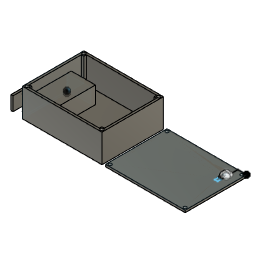
Cadeadov1.0 v4-Tampa (Autodesk Fusion 360 design; units mm, degrees)
Autodesk Fusion 360 part; units mm, degrees
note: some values were not read from the file. Set by a fixed rule: which sketch regions a step uses.
sketch "Sketch1" plane through (0, 0, 0) normal (0, 0, 1) x (1, 0, 0)
  line L0 (0, 0) -> (110, 0)
  line L1 (110, 0) -> (110, 85)
  line L2 (110, 85) -> (0, 85)
  line L3 (0, 85) -> (0, 0)
  dimension "d1" = 110
  dimension "d2" = 85
  constraint horizontal L0
  constraint vertical L1
  constraint horizontal L2
  constraint vertical L3
  constraint coincident L0.start L3.end
  measures "d1" distance of L0.start L0.end
  measures "d2" distance of L0.start L2.end
extrude "Extrude1" add sketch "Sketch1" along normal blind 3 makes body 1
sketch "Sketch2" plane through (0, 0, 3) normal (0, 0, 1) x (-1, 0, 0)
  line L0 (0, -85) -> (0, 0)
  line L1 (0, 0) -> (-110, 0)
  line L2 (-110, 0) -> (-110, -85)
  line L3 (-110, -85) -> (0, -85)
  line L4 (0, 0) -> (-6.5, 0)
  line L5 (-6.5, 0) -> (-6.5, -6.5)
  line L6 (-6.5, -6.5) -> (0, -6.5)
  line L7 (0, -6.5) -> (0, 0)
  line L8 (0, -85) -> (-6.5, -85)
  line L9 (-6.5, -85) -> (-6.5, -78.5)
  line L10 (-6.5, -78.5) -> (0, -78.5)
  line L11 (0, -78.5) -> (0, -85)
  line L12 (-110, -85) -> (-103.5, -85)
  line L13 (-103.5, -85) -> (-103.5, -78.5)
  line L14 (-103.5, -78.5) -> (-110, -78.5)
  line L15 (-110, -78.5) -> (-110, -85)
  line L16 (-110, 0) -> (-103.5, 0)
  line L17 (-103.5, 0) -> (-103.5, -6.5)
  line L18 (-103.5, -6.5) -> (-110, -6.5)
  line L19 (-110, -6.5) -> (-110, 0)
  line L20 (-6.5, 0) -> (-103.5, 0)
  line L21 (-103.5, 0) -> (-103.5, -3)
  line L22 (-103.5, -3) -> (-6.5, -3)
  line L23 (-6.5, -3) -> (-6.5, 0)
  line L24 (-110, -6.5) -> (-107, -6.5)
  line L25 (-107, -6.5) -> (-107, -78.5)
  line L26 (-107, -78.5) -> (-110, -78.5)
  line L27 (-110, -78.5) -> (-110, -6.5)
  line L28 (-103.5, -85) -> (-6.5, -85)
  line L29 (-6.5, -85) -> (-6.5, -82)
  line L30 (-6.5, -82) -> (-103.5, -82)
  line L31 (-103.5, -82) -> (-103.5, -85)
  line L32 (0, -78.5) -> (-3, -78.5)
  line L33 (-3, -78.5) -> (-3, -6.5)
  line L34 (-3, -6.5) -> (0, -6.5)
  line L35 (0, -6.5) -> (0, -78.5)
  dimension "d5" = 6.5
  dimension "d6" = 6.5
  dimension "d7" = 6.5
  dimension "d8" = 6.5
  dimension "d9" = 6.5
  dimension "d10" = 6.5
  dimension "d11" = 6.5
  dimension "d12" = 6.5
  dimension "d13" = 97
  dimension "d14" = 3
  dimension "d15" = 3
  dimension "d16" = 72
  dimension "d17" = 3
  dimension "d18" = 3
  constraint horizontal L4
  constraint vertical L5
  constraint horizontal L6
  constraint vertical L7
  constraint coincident L0.end L1.start
  constraint horizontal L8
  constraint vertical L9
  constraint horizontal L10
  constraint vertical L11
  constraint coincident L0.start L3.end
  constraint horizontal L12
  constraint vertical L13
  constraint horizontal L14
  constraint vertical L15
  constraint coincident L2.end L3.start
  constraint horizontal L16
  constraint vertical L17
  constraint horizontal L18
  constraint vertical L19
  constraint coincident L1.end L2.start
  constraint horizontal L20
  constraint vertical L21
  constraint horizontal L22
  constraint vertical L23
  constraint horizontal L24
  constraint vertical L25
  constraint horizontal L26
  constraint vertical L27
  constraint horizontal L28
  constraint vertical L29
  constraint horizontal L30
  constraint vertical L31
  constraint horizontal L32
  constraint vertical L33
  constraint horizontal L34
  constraint vertical L35
  constraint coincident L6 L33.end
  measures "d5" distance of L0.end L4.end
  measures "d6" distance of L0.end L6.end
  measures "d7" distance of L0.start L8.end
  measures "d8" distance of L0.start L10.end
  measures "d9" distance of L2.end L12.end
  measures "d10" distance of L2.end L14.end
  measures "d11" distance of L1.end L16.end
  measures "d12" distance of L1.end L18.end
  measures "d13" distance of L4.end L16.end
  measures "d14" distance of L4.end L22.end
  measures "d15" distance of L18.end L24.end
  measures "d16" distance of L18.end L14.end
  measures "d17" distance of L12.end L30.end
  measures "d18" distance of L10.end L32.end
extrude "Extrude2" add sketch "Sketch2" along normal blind 36 contours L0 L3 L8 L9 L10 L11 L29 L32 | L0 L6 L10 L32 L33 L34 L35 | L3 L9 L13 L28 L29 L30 L31 | L0 L1 L4 L5 L6 L7 L23 L34 | L2 L3 L12 L13 L14 L15 L26 L31 | L1 L5 L17 L20 L21 L22 L23 | L2 L14 L18 L24 L25 L26 L27 | L1 L2 L16 L17 L18 L19 L21 L24 bodies 1
sketch "Sketch3" plane through (0, 0, 3) normal (0, 0, 1) x (-1, 0, 0)
  line L0 (-6.5, -78.5) -> (-3, -78.5)
  line L1 (-3, -78.5) -> (-3, -6.5)
  line L2 (-3, -6.5) -> (-6.5, -6.5)
  line L3 (-6.5, -6.5) -> (-6.5, -3)
  line L4 (-6.5, -3) -> (-103.5, -3)
  line L5 (-103.5, -3) -> (-103.5, -6.5)
  line L6 (-103.5, -6.5) -> (-107, -6.5)
  line L7 (-107, -6.5) -> (-107, -78.5)
  line L8 (-107, -78.5) -> (-103.5, -78.5)
  line L9 (-103.5, -78.5) -> (-103.5, -82)
  line L10 (-103.5, -82) -> (-6.5, -82)
  line L11 (-6.5, -82) -> (-6.5, -78.5)
  line L12 (-6.5, -3) -> (-33.5, -3)
  line L13 (-6.5, -6.5) -> (-6.5, -61.5)
  line L14 (-6.5, -61.5) -> (-1.333, -61.5)
  line L15 (-3, -61.5) -> (-36.5, -61.5)
  line L16 (-36.5, -61.5) -> (-36.5, -64.5)
  line L17 (-36.5, -64.5) -> (-3, -64.5)
  line L18 (-3, -64.5) -> (-3, -61.5)
  line L19 (-36.5, -64.5) -> (-33.5, -64.5)
  line L20 (-33.5, -64.5) -> (-33.5, -3)
  line L21 (-33.5, -3) -> (-36.5, -3)
  line L22 (-36.5, -3) -> (-36.5, -64.5)
  dimension "d21" = 27
  dimension "d22" = 55
  dimension "d23" = 33.5
  dimension "d24" = 3
  constraint coincident L3.end L4.start
  constraint perpendicular L3 L12
  constraint coincident L2.end L3.start
  constraint perpendicular L2 L13
  constraint perpendicular L1 L14
  constraint horizontal L15
  constraint vertical L16
  constraint horizontal L17
  constraint vertical L18
  constraint coincident L14 L15.start
  constraint coincident L1 L15.start
  constraint horizontal L19
  constraint vertical L20
  constraint horizontal L21
  constraint vertical L22
  measures "d21" distance of L3.end L12.end
  measures "d22" distance of L2.end L13.end
  measures "d23" distance of L15.start L15.end
  measures "d24" distance of L15.start L17.end
extrude "Extrude3" add sketch "Sketch3" along normal blind 20.5 contours L1 L14 L15 L17 L18 L20 | L15 L16 L17 L19 L20 L22 | L4 L15 L20 L21 L22 bodies 1
sketch "Sketch4" plane through (0, 0, 23.5) normal (0, 0, 1) x (-1, 0, 0)
  line L0 (-36.5, -3) -> (-36.5, -64.5)
  line L1 (-36.5, -64.5) -> (-3, -64.5)
  line L2 (-3, -64.5) -> (-3, -61.5)
  line L3 (-3, -61.5) -> (-33.5, -61.5)
  line L4 (-33.5, -61.5) -> (-33.5, -3)
  line L5 (-33.5, -3) -> (-36.5, -3)
  line L6 (-3, -64.5) -> (-36.5, -64.5)
  line L7 (-36.5, -64.5) -> (-36.5, -3)
  line L8 (-36.5, -3) -> (-3, -3)
  line L9 (-3, -3) -> (-3, -64.5)
  constraint horizontal L6
  constraint vertical L7
  constraint horizontal L8
  constraint vertical L9
  constraint coincident L0.start L5.end
  constraint coincident L1.end L2.start
sketch "Sketch5" plane through (0, 0, 23.5) normal (0, 0, 1) x (1, 0, 0)
sketch "Sketch6" plane through (0, 0, 23.5) normal (0, 0, 1) x (1, 0, 0)
sketch "Sketch7" plane through (0, 0, 23.5) normal (0, 0, 1) x (-1, 0, 0)
extrude "Extrude4" add sketch "Sketch4" along normal blind 3 contours L0 L1 L2 L3 L4 L5 L6 L7 L8 L9 bodies 1
sketch "Sketch8" plane through (0, 61.5, 0) normal (0, -1, 0) x (1, 0, 0)
  line L0 (3, 3) -> (33.5, 3)
  line L1 (33.5, 3) -> (33.5, 26.5)
  line L2 (33.5, 26.5) -> (3, 26.5)
  line L3 (3, 26.5) -> (3, 3)
  line L4 (3, 26.5) -> (33.5, 26.5)
  line L5 (33.5, 26.5) -> (33.5, 23.5)
  line L6 (33.5, 23.5) -> (3, 23.5)
  line L7 (3, 23.5) -> (3, 26.5)
  dimension "d29" = 3
  constraint horizontal L4
  constraint vertical L5
  constraint horizontal L6
  constraint vertical L7
  constraint coincident L2.end L3.start
  measures "d29" distance of L2.end L6.end
extrude "Extrude5" add sketch "Sketch8" along normal blind 55 contours L1 L2 L3 L4 L5 L6 L7 bodies 1
sketch "Sketch9" plane through (33.5, 0, 0) normal (-1, 0, 0) x (0, -1, 0)
  line L0 (-6.5, 23.5) -> (-61.5, 23.5)
  line L1 (-61.5, 23.5) -> (-61.5, 3)
  line L2 (-61.5, 3) -> (-3, 3)
  line L3 (-3, 3) -> (-3, 26.5)
  line L4 (-3, 26.5) -> (-6.5, 26.5)
  line L5 (-6.5, 26.5) -> (-6.5, 23.5)
  line L6 (-6.5, 26.5) -> (-3, 26.5)
  line L7 (-3, 26.5) -> (-3, 23.5)
  line L8 (-3, 23.5) -> (-6.5, 23.5)
  line L9 (-6.5, 23.5) -> (-6.5, 26.5)
  dimension "d32" = 3
  constraint horizontal L6
  constraint vertical L7
  constraint horizontal L8
  constraint vertical L9
  constraint coincident L4.end L5.start
  measures "d32" distance of L4.end L0.start
extrude "Extrude6" add sketch "Sketch9" along normal blind 27 contours L3 L4 L5 L6 L7 L8 L9 bodies 1
sketch "Sketch10" plane through (0, 0, 0) normal (-1, 0, 0) x (0, -1, 0)
  line L0 (-85, 0) -> (0, 0)
  line L1 (0, 0) -> (0, 39)
  line L2 (0, 39) -> (-85, 39)
  line L3 (-85, 39) -> (-85, 0)
  line L4 (0, 0) -> (-6.5, 0)
  line L5 (-6.5, 0) -> (-6.5, 3)
  line L6 (-6.5, 3) -> (-6.5, 23.5)
  line L7 (-6.5, 23.5) -> (-61.5, 23.5)
  line L8 (-61.5, 23.5) -> (-61.5, 3)
  line L9 (-61.5, 3) -> (-6.5, 3)
  dimension "d35" = 6.5
  dimension "d36" = 3
  dimension "d37" = 20.5
  dimension "d38" = 55
  constraint coincident L0.end L1.start
  constraint perpendicular L1 L4
  constraint perpendicular L4 L5
  constraint perpendicular L0 L6
  constraint perpendicular L6 L7
  constraint perpendicular L0 L8
  constraint perpendicular L5 L9
  measures "d35" distance of L0.end L4.end
  measures "d36" distance of L4.end L5.end
  measures "d37" distance of L5.end L6.end
  measures "d38" distance of L6.end L7.end
extrude "Extrude7" cut sketch "Sketch10" against normal blind 3 contours L6 L7 L8 L9 bodies 1
sketch "Sketch11" plane through (0, 0, 39) normal (0, 0, 1) x (-1, 0, 0)
  line L0 (-6.5, -78.5) -> (-6.5, -82)
  line L1 (-6.5, -82) -> (-103.5, -82)
  line L2 (-103.5, -82) -> (-103.5, -78.5)
  line L3 (-103.5, -78.5) -> (-107, -78.5)
  line L4 (-107, -78.5) -> (-107, -6.5)
  line L5 (-107, -6.5) -> (-103.5, -6.5)
  line L6 (-103.5, -6.5) -> (-103.5, -3)
  line L7 (-103.5, -3) -> (-6.5, -3)
  line L8 (-6.5, -3) -> (-6.5, -6.5)
  line L9 (-6.5, -6.5) -> (-3, -6.5)
  line L10 (-3, -6.5) -> (-3, -78.5)
  line L11 (-3, -78.5) -> (-6.5, -78.5)
  line L12 (0, 0) -> (-110, 0)
  line L13 (-110, 0) -> (-110, -85)
  line L14 (-110, -85) -> (0, -85)
  line L15 (0, -85) -> (0, 0)
  line L16 (0, -78.5) -> (-3.25, -78.5)
  line L17 (-3.25, -78.5) -> (-3.25, -81.75)
  circle A0 centre (-3.25, -81.75) radius 2.2
  line L18 (0, 0) -> (-3.25, 0)
  line L19 (-3.25, 0) -> (-3.25, -3.25)
  circle A1 centre (-3.25, -3.25) radius 2.2
  line L20 (-110, 0) -> (-106.75, 0)
  line L21 (-106.75, 0) -> (-106.75, -3.25)
  circle A2 centre (-106.75, -3.25) radius 2.2
  line L22 (-110, -85) -> (-106.75, -85)
  line L23 (-106.75, -85) -> (-106.75, -81.75)
  circle A3 centre (-106.75, -81.75) radius 2.2
  dimension "d41" = 3.25
  dimension "d42" = 3.25
  dimension "d43" = 4.4
  dimension "d44" = 3.25
  dimension "d45" = 3.25
  dimension "d46" = 4.4
  dimension "d47" = 3.25
  dimension "d48" = 3.25
  dimension "d49" = 4.4
  dimension "d50" = 3.25
  dimension "d51" = 3.25
  dimension "d52" = 4.4
  constraint coincident L15 L16.start
  constraint perpendicular L10 L16
  constraint perpendicular L14 L17
  constraint coincident L17.end A0.centre
  constraint coincident L12.start L15.end
  constraint perpendicular L15 L18
  constraint perpendicular L12 L19
  constraint coincident L19.end A1.centre
  constraint coincident L12.end L13.start
  constraint perpendicular L13 L20
  constraint perpendicular L20 L21
  constraint coincident L21.end A2.centre
  constraint coincident L13.end L14.start
  constraint perpendicular L13 L22
  constraint perpendicular L22 L23
  constraint coincident L23.end A3.centre
  measures "d41" distance of L16.start L16.end
  measures "d42" distance of L16.end L17.end
  measures "d43" diameter of A0
  measures "d44" distance of L12.start L18.end
  measures "d45" distance of L18.end L19.end
  measures "d46" diameter of A1
  measures "d47" distance of L12.end L20.end
  measures "d48" distance of L20.end L21.end
  measures "d49" diameter of A2
  measures "d50" distance of L13.end L22.end
  measures "d51" distance of L22.end L23.end
  measures "d52" diameter of A3
extrude "Extrude8" cut sketch "Sketch11" against normal blind 15 contours A0 | A1 | A2 | A3 bodies 1
sketch "Sketch12" plane through (0, 0, 0) normal (0, 0, 1) x (1, 0, 0)
  line L0 (115, 0) -> (225, 0)
  line L1 (225, 0) -> (225, 85)
  line L2 (225, 85) -> (115, 85)
  line L3 (115, 85) -> (115, 0)
  dimension "d55" = 110
  dimension "d56" = 85
  constraint horizontal L0
  constraint vertical L1
  constraint horizontal L2
  constraint vertical L3
  measures "d55" distance of L0.start L0.end
  measures "d56" distance of L0.start L2.end
extrude "Extrude9" add sketch "Sketch12" along normal blind 3 separate body makes body 2
sketch "Sketch13" plane through (0, 0, 3) normal (0, 0, 1) x (-1, 0, 0)
  line L0 (-115, -85) -> (-115, 0)
  line L1 (-115, 0) -> (-225, 0)
  line L2 (-225, 0) -> (-225, -85)
  line L3 (-225, -85) -> (-115, -85)
  line L4 (-115, 0) -> (-118.25, 0)
  line L5 (-118.25, 0) -> (-118.25, -3.25)
  circle A0 centre (-118.25, -3.25) radius 2.2
  line L6 (-115, -85) -> (-118.25, -85)
  line L7 (-118.25, -85) -> (-118.25, -81.75)
  circle A1 centre (-118.25, -81.75) radius 2.2
  line L8 (-225, -85) -> (-221.75, -85)
  line L9 (-221.75, -85) -> (-221.75, -81.75)
  circle A2 centre (-221.75, -81.75) radius 2.2
  line L10 (-225, 0) -> (-221.75, 0)
  line L11 (-221.75, 0) -> (-221.75, -3.25)
  circle A3 centre (-221.75, -3.25) radius 2.2
  circle A4 centre (-118.25, -81.75) radius 2.1
  circle A5 centre (-221.75, -81.75) radius 2.1
  circle A6 centre (-221.75, -3.25) radius 2.1
  circle A7 centre (-118.25, -3.25) radius 2.1
  dimension "d59" = 3.25
  dimension "d60" = 3.25
  dimension "d61" = 4.4
  dimension "d62" = 3.25
  dimension "d63" = 3.25
  dimension "d64" = 4.4
  dimension "d65" = 3.25
  dimension "d66" = 3.25
  dimension "d67" = 4.4
  dimension "d68" = 3.25
  dimension "d69" = 3.25
  dimension "d70" = 4.4
  dimension "d71" = 4.2
  dimension "d72" = 4.2
  dimension "d73" = 4.2
  dimension "d74" = 4.2
  constraint coincident L0.end L1.start
  constraint perpendicular L0 L4
  constraint perpendicular L4 L5
  constraint coincident L5.end A0.centre
  constraint coincident L0.start L3.end
  constraint perpendicular L0 L6
  constraint perpendicular L6 L7
  constraint coincident L7.end A1.centre
  constraint coincident L2.end L3.start
  constraint perpendicular L2 L8
  constraint perpendicular L8 L9
  constraint coincident L9.end A2.centre
  constraint coincident L1.end L2.start
  constraint perpendicular L2 L10
  constraint perpendicular L10 L11
  constraint coincident L11.end A3.centre
  constraint concentric A1 A4
  constraint concentric A2 A5
  constraint concentric A3 A6
  constraint concentric A0 A7
  measures "d59" distance of L0.end L4.end
  measures "d60" distance of L4.end L5.end
  measures "d61" diameter of A0
  measures "d62" distance of L0.start L6.end
  measures "d63" distance of L6.end L7.end
  measures "d64" diameter of A1
  measures "d65" distance of L2.end L8.end
  measures "d66" distance of L8.end L9.end
  measures "d67" diameter of A2
  measures "d68" distance of L1.end L10.end
  measures "d69" distance of L10.end L11.end
  measures "d70" diameter of A3
  measures "d71" diameter of A4
  measures "d72" diameter of A5
  measures "d73" diameter of A6
  measures "d74" diameter of A7
extrude "Extrude10" cut sketch "Sketch13" against normal blind 3 contours A4 | A5 | A6 | A7 bodies 2
sketch "Sketch14" plane through (0, 61.5, 0) normal (0, -1, 0) x (1, 0, 0)
  line L0 (33.5, 23.5) -> (0, 23.5)
  line L1 (0, 23.5) -> (0, 3)
  line L2 (0, 3) -> (33.5, 3)
  line L3 (33.5, 3) -> (33.5, 23.5)
  line L4 (0, 3) -> (3, 3)
  line L5 (3, 3) -> (3, 6)
  line L6 (3, 6) -> (0, 6)
  line L7 (0, 6) -> (0, 3)
  constraint horizontal L4
  constraint vertical L5
  constraint horizontal L6
  constraint vertical L7
  constraint coincident L1.end L2.start
sketch "Sketch15" plane through (0, 61.5, 0) normal (0, -1, 0) x (1, 0, 0)
  line L0 (0, 6) -> (3, 6)
  line L1 (3, 6) -> (3, 9)
  line L2 (3, 9) -> (0, 9)
  line L3 (0, 9) -> (0, 6)
  constraint horizontal L0
  constraint vertical L1
  constraint horizontal L2
  constraint vertical L3
extrude "Extrude11" cut sketch "Sketch15" against normal blind 3 bodies 1
sketch "Sketch16" plane through (16.75, 61.5, 13.25) normal (0, -1, 0) x (1, 0, 0)
sketch "Sketch17" plane through (16.75, 61.5, 13.25) normal (0, -1, 0) x (1, 0, 0)
sketch "Sketch18" plane through (0, 0, 0) normal (-1, 0, 0) x (0, -1, 0)
  line L0 (-85, 0) -> (0, 0)
  line L1 (0, 0) -> (0, 39)
  line L2 (0, 39) -> (-85, 39)
  line L3 (-85, 39) -> (-85, 0)
  line L4 (-61.5, 6) -> (-64.5, 6)
  line L5 (-64.5, 6) -> (-64.5, 9)
  line L6 (-64.5, 9) -> (-61.5, 9)
  line L7 (-61.5, 9) -> (-61.5, 23.5)
  line L8 (-61.5, 23.5) -> (-6.5, 23.5)
  line L9 (-6.5, 23.5) -> (-6.5, 3)
  line L10 (-6.5, 3) -> (-61.5, 3)
  line L11 (-61.5, 3) -> (-61.5, 6)
  line L12 (-64.5, 9) -> (-61.5, 9)
  line L13 (-61.5, 9) -> (-61.5, 12)
  line L14 (-61.5, 12) -> (-64.5, 12)
  line L15 (-64.5, 12) -> (-64.5, 9)
  line L16 (-61.5, 12) -> (-64.5, 12)
  line L17 (-64.5, 12) -> (-64.5, 15)
  line L18 (-64.5, 15) -> (-61.5, 15)
  line L19 (-61.5, 15) -> (-61.5, 12)
  constraint horizontal L12
  constraint vertical L13
  constraint horizontal L14
  constraint vertical L15
  constraint coincident L7 L13.end
  constraint coincident L5.end L6.start
  constraint horizontal L16
  constraint vertical L17
  constraint horizontal L18
  constraint vertical L19
extrude "Extrude12" cut sketch "Sketch18" against normal blind 3 contours L7 L14 L16 L17 L18 L19 bodies 1
sketch "Sketch19" plane through (0, 0, 0) normal (-1, 0, 0) x (0, -1, 0)
  line L0 (-64.5, 15) -> (-61.5, 15)
  line L1 (-61.5, 15) -> (-61.5, 23.5)
  line L2 (-61.5, 23.5) -> (-6.5, 23.5)
  line L3 (-6.5, 23.5) -> (-6.5, 3)
  line L4 (-6.5, 3) -> (-61.5, 3)
  line L5 (-61.5, 3) -> (-61.5, 6)
  line L6 (-61.5, 6) -> (-64.5, 6)
  line L7 (-64.5, 6) -> (-64.5, 9)
  line L8 (-64.5, 9) -> (-61.5, 9)
  line L9 (-61.5, 9) -> (-61.5, 12)
  line L10 (-61.5, 12) -> (-64.5, 12)
  line L11 (-64.5, 12) -> (-64.5, 15)
  line L12 (-85, 0) -> (0, 0)
  line L13 (0, 0) -> (0, 39)
  line L14 (0, 39) -> (-85, 39)
  line L15 (-85, 39) -> (-85, 0)
  line L16 (-61.5, 15) -> (-64.5, 15)
  line L17 (-64.5, 15) -> (-64.5, 18)
  line L18 (-64.5, 18) -> (-61.5, 18)
  line L19 (-61.5, 18) -> (-61.5, 15)
  line L20 (-61.5, 18) -> (-64.5, 18)
  line L21 (-64.5, 18) -> (-64.5, 21)
  line L22 (-64.5, 21) -> (-61.5, 21)
  line L23 (-61.5, 21) -> (-61.5, 18)
  dimension "d81" = 3
  dimension "d82" = 3
  dimension "d83" = 3
  dimension "d84" = 3
  constraint horizontal L16
  constraint vertical L17
  constraint horizontal L18
  constraint vertical L19
  constraint coincident L0.end L1.start
  constraint horizontal L20
  constraint vertical L21
  constraint horizontal L22
  constraint vertical L23
  measures "d81" distance of L0.end L0.start
  measures "d82" distance of L0.end L18.end
  measures "d83" distance of L18.end L17.end
  measures "d84" distance of L18.end L22.end
extrude "Extrude13" cut sketch "Sketch19" against normal blind 3 contours L1 L18 L20 L21 L22 L23 bodies 1
sketch "Sketch20" plane through (0, 0, 0) normal (0, 0, 1) x (1, 0, 0)
  line L0 (-15, 2) -> (-18, 2)
  line L1 (-18, 2) -> (-18, 60)
  line L2 (-18, 60) -> (-15, 60)
  line L3 (-15, 60) -> (-15, 2)
  line L4 (-18, 60) -> (-15, 60)
  line L5 (-15, 60) -> (-15, 57)
  line L6 (-15, 57) -> (-18, 57)
  line L7 (-18, 57) -> (-18, 60)
  circle A0 centre (-16.5, 58.5) radius 1.5
  dimension "d87" = 3
  dimension "d88" = 58
  dimension "d89" = 3
  dimension "d90" = 3
  constraint horizontal L0
  constraint vertical L1
  constraint horizontal L2
  constraint vertical L3
  constraint horizontal L4
  constraint vertical L5
  constraint horizontal L6
  constraint vertical L7
  constraint tangent L3 A0
  measures "d87" distance of L0.start L0.end
  measures "d88" distance of L0.start L2.end
  measures "d89" distance of L1.end L2.end
  measures "d90" distance of L1.end L6.end
extrude "Extrude14" add sketch "Sketch20" along normal blind 20 separate body contours L0 L1 L3 L6 | L3 L5 L6 A0 | L1 L6 L7 A0 | A0 makes body 3
extrude "Extrude15" cut 1 faces at (-17, 38.6667, 20) along direction (0, 0, -1) blind 1 on bodies 3 bodies 3
sketch "Sketch21" plane through (-18, 0, 0) normal (-1, 0, 0) x (0, -1, 0)
  line L0 (-2, 19) -> (-58.5, 19)
  line L1 (-58.5, 19) -> (-58.5, 0)
  line L2 (-58.5, 0) -> (-2, 0)
  line L3 (-2, 0) -> (-2, 19)
  line L4 (-60, 0) -> (-57, 0)
  line L5 (-57, 0) -> (-57, 2.25)
  line L6 (-57, 2.25) -> (-60, 2.25)
  line L7 (-60, 2.25) -> (-60, 0)
  line L8 (-57, 2.25) -> (-60, 2.25)
  line L9 (-60, 2.25) -> (-60, 5.15)
  line L10 (-60, 5.15) -> (-57, 5.15)
  line L11 (-57, 5.15) -> (-57, 2.25)
  dimension "d95" = 3
  dimension "d96" = 2.25
  dimension "d97" = 2.9
  constraint horizontal L4
  constraint vertical L5
  constraint horizontal L6
  constraint vertical L7
  constraint horizontal L8
  constraint vertical L9
  constraint horizontal L10
  constraint vertical L11
  measures "d95" distance of L4.start L4.end
  measures "d96" distance of L4.start L6.end
  measures "d97" distance of L5.end L10.end
sketch "Sketch22" plane through (-18, 30.25, 9.5) normal (-1, 0, 0) x (0, -1, 0)
extrude "Extrude16" cut sketch "Sketch21" against normal blind 4 contours L1 L2 L4 L5 L6 L8 | L1 L4 L6 L7 L8 bodies 3
sketch "Sketch23" plane through (-18, 0, 0) normal (-1, 0, 0) x (0, -1, 0)
  line L0 (-57, 2.25) -> (-57, 0)
  line L1 (-57, 0) -> (-2, 0)
  line L2 (-2, 0) -> (-2, 19)
  line L3 (-2, 19) -> (-58.5, 19)
  line L4 (-58.5, 19) -> (-58.5, 2.25)
  line L5 (-58.5, 2.25) -> (-57, 2.25)
  line L6 (-57, 2.25) -> (-60, 2.25)
  line L7 (-60, 2.25) -> (-60, 5.15)
  line L8 (-60, 5.15) -> (-57, 5.15)
  line L9 (-57, 5.15) -> (-57, 2.25)
  line L10 (-57, 5.15) -> (-59.9423, 5.15)
  line L11 (-59.9423, 5.15) -> (-59.9423, 8.3)
  line L12 (-59.9423, 8.3) -> (-57, 8.3)
  line L13 (-57, 8.3) -> (-57, 5.15)
  line L14 (-57, 8.3) -> (-60, 8.3)
  line L15 (-60, 8.3) -> (-60, 11.2)
  line L16 (-60, 11.2) -> (-57, 11.2)
  line L17 (-57, 11.2) -> (-57, 8.3)
  line L18 (-57, 11.2) -> (-60, 11.2)
  line L19 (-60, 11.2) -> (-60, 14.25)
  line L20 (-60, 14.25) -> (-57, 14.25)
  line L21 (-57, 14.25) -> (-57, 11.2)
  line L22 (-57, 14.25) -> (-60, 14.25)
  line L23 (-60, 14.25) -> (-60, 17.15)
  line L24 (-60, 17.15) -> (-57, 17.15)
  line L25 (-57, 17.15) -> (-57, 14.25)
  line L26 (-57, 17.15) -> (-60, 17.15)
  line L27 (-60, 17.15) -> (-60, 19)
  line L28 (-60, 19) -> (-57, 19)
  line L29 (-57, 19) -> (-57, 17.15)
  dimension "d100" = 3
  dimension "d101" = 2.9
  dimension "d102" = 3.15
  dimension "d103" = 3
  dimension "d104" = 2.9
  dimension "d105" = 3
  dimension "d106" = 3.05
  dimension "d107" = 3
  dimension "d108" = 2.9
  constraint horizontal L6
  constraint vertical L7
  constraint horizontal L8
  constraint vertical L9
  constraint coincident L0.start L5.end
  constraint horizontal L10
  constraint vertical L11
  constraint horizontal L12
  constraint vertical L13
  constraint horizontal L14
  constraint vertical L15
  constraint horizontal L16
  constraint vertical L17
  constraint horizontal L18
  constraint vertical L19
  constraint horizontal L20
  constraint vertical L21
  constraint horizontal L22
  constraint vertical L23
  constraint horizontal L24
  constraint vertical L25
  constraint horizontal L26
  constraint vertical L27
  constraint horizontal L28
  constraint vertical L29
  measures "d100" distance of L0.start L6.end
  measures "d101" distance of L0.start L8.end
  measures "d102" distance of L8.end L12.end
  measures "d103" distance of L12.end L14.end
  measures "d104" distance of L12.end L16.end
  measures "d105" distance of L16.end L15.end
  measures "d106" distance of L16.end L20.end
  measures "d107" distance of L20.end L19.end
  measures "d108" distance of L20.end L24.end
extrude "Extrude17" cut sketch "Sketch23" against normal blind 4 contours L4 L8 L10 L12 L13 L14 | L4 L8 L10 L11 L12 L14 | L4 L16 L18 L20 L21 L22 | L3 L4 L24 L26 L28 L29 | L4 L16 L18 L19 L20 L22 | L4 L24 L26 L27 L28 bodies 3
extrude "Extrude18" cut 1 faces at (-17, 57, 7.25) along direction (0, 1, 0) blind 3.5 on bodies 3 bodies 3
sketch "Sketch24" plane through (0, 0, 17.15) normal (0, 0, 1) x (-1, 0, 0)
  arc A0 (15, -58.5) -> (18, -58.5) centre (16.5, -58.5) ccw
  line L0 (18, -58.5) -> (18, -57)
  line L1 (18, -57) -> (15, -57)
  line L2 (15, -57) -> (15, -58.5)
  line L3 (15, -57) -> (18, -57)
  line L4 (18, -57) -> (18, -60)
  line L5 (18, -60) -> (15, -60)
  line L6 (15, -60) -> (15, -57)
  circle A1 centre (16.5, -58.5) radius 0.65
  dimension "d113" = 3
  dimension "d114" = 1.3
  constraint horizontal L3
  constraint vertical L4
  constraint horizontal L5
  constraint vertical L6
  constraint coincident L1.end L2.start
  constraint concentric A0 A1
  measures "d113" distance of L1.end L0.end
  measures "d114" diameter of A1
extrude "Extrude19" cut sketch "Sketch24" against normal blind 17 contours A1 bodies 3
sketch "Sketch25" plane through (0, 0, 0) normal (-1, 0, 0) x (0, -1, 0)
  line L0 (-64.5, 21) -> (-61.5, 21)
  line L1 (-61.5, 21) -> (-61.5, 23.5)
  line L2 (-61.5, 23.5) -> (-6.5, 23.5)
  line L3 (-6.5, 23.5) -> (-6.5, 3)
  line L4 (-6.5, 3) -> (-61.5, 3)
  line L5 (-61.5, 3) -> (-61.5, 6)
  line L6 (-61.5, 6) -> (-64.5, 6)
  line L7 (-64.5, 6) -> (-64.5, 9)
  line L8 (-64.5, 9) -> (-61.5, 9)
  line L9 (-61.5, 9) -> (-61.5, 12)
  line L10 (-61.5, 12) -> (-64.5, 12)
  line L11 (-64.5, 12) -> (-64.5, 15)
  line L12 (-64.5, 15) -> (-61.5, 15)
  line L13 (-61.5, 15) -> (-61.5, 18)
  line L14 (-61.5, 18) -> (-64.5, 18)
  line L15 (-64.5, 18) -> (-64.5, 21)
  line L16 (-85, 0) -> (0, 0)
  line L17 (0, 0) -> (0, 39)
  line L18 (0, 39) -> (-85, 39)
  line L19 (-85, 39) -> (-85, 0)
  line L20 (-61.5, 3) -> (-61.5, 0)
  constraint coincident L4.end L5.start
  constraint coincident L16 L20.end
  constraint perpendicular L16 L20
sketch "Sketch26" plane through (0, 0, 0) normal (0, 0, -1) x (1, 0, 0)
  line L0 (0, 0) -> (0, -85)
  line L1 (0, -85) -> (110, -85)
  line L2 (110, -85) -> (110, 0)
  line L3 (110, 0) -> (0, 0)
  line L4 (0, -61.5) -> (3, -61.5)
  line L5 (3, -61.5) -> (3, -64.5)
  line L6 (3, -64.5) -> (0, -64.5)
  line L7 (0, -64.5) -> (0, -61.5)
  line L8 (3, -61.5) -> (1.5, -61.5)
  line L9 (1.5, -61.5) -> (1.5, -63)
  circle A0 centre (1.5, -63) radius 0.65
  dimension "d117" = 3
  dimension "d118" = 3
  dimension "d119" = 1.3
  constraint coincident L0 L4.start
  constraint perpendicular L0 L4
  constraint perpendicular L4 L5
  constraint coincident L0 L6.end
  constraint perpendicular L0 L6
  constraint midpoint L4 L8.end
  constraint perpendicular L4 L9
  constraint coincident L9.end A0.centre
  measures "d117" distance of L4.start L4.end
  measures "d118" distance of L4.end L5.end
  measures "d119" diameter of A0
extrude "Extrude20" cut sketch "Sketch26" against normal blind 23 contours A0 bodies 1
sketch "Sketch27" plane through (0, 0, 0) normal (0, 0, 1) x (1, 0, 0)
  circle A0 centre (-9, 9) radius 0.575
  dimension "d122" = 1.15
  measures "d122" diameter of A0
extrude "Extrude21" add sketch "Sketch27" along normal blind 21 separate body makes body 4
sketch "Sketch28" plane through (0, 0, 0) normal (0, 0, 1) x (1, 0, 0)
  circle A0 centre (-8, 17) radius 0.64
  dimension "d125" = 1.28
  measures "d125" diameter of A0
extrude "Extrude22" add sketch "Sketch28" along normal blind 1.9 separate body makes body 5
sketch "Sketch29" plane through (0, 0, 3) normal (0, 0, 1) x (-1, 0, 0)
  circle A0 centre (-118.25, -81.75) radius 2.1
  circle A1 centre (-221.75, -81.75) radius 2.1
  circle A2 centre (-118.25, -3.25) radius 2.1
  circle A3 centre (-221.75, -3.25) radius 2.1
  line L0 (-115, -85) -> (-115, 0)
  line L1 (-115, 0) -> (-225, 0)
  line L2 (-225, 0) -> (-225, -85)
  line L3 (-225, -85) -> (-115, -85)
  line L4 (-225, -85) -> (-213, -85)
  line L5 (-213, -85) -> (-213, -73)
  line L6 (-213, -73) -> (-209, -73)
  line L7 (-209, -73) -> (-209, -69)
  line L8 (-209, -69) -> (-213, -69)
  line L9 (-213, -69) -> (-213, -73)
  line L10 (-209, -69) -> (-213, -69)
  line L11 (-213, -69) -> (-213, -61)
  line L12 (-213, -61) -> (-209, -61)
  line L13 (-209, -61) -> (-209, -69)
  line L14 (-209, -61) -> (-209, -65)
  line L15 (-209, -65) -> (-213, -65)
  dimension "d128" = 12
  dimension "d129" = 12
  dimension "d130" = 4
  dimension "d131" = 4
  dimension "d132" = 4
  dimension "d133" = 8
  constraint coincident L2.end L3.start
  constraint perpendicular L2 L4
  constraint perpendicular L4 L5
  constraint horizontal L6
  constraint vertical L7
  constraint horizontal L8
  constraint vertical L9
  constraint horizontal L10
  constraint vertical L11
  constraint horizontal L12
  constraint vertical L13
  constraint midpoint L13 L14.end
  constraint midpoint L11 L15.end
  measures "d128" distance of L2.end L4.end
  measures "d129" distance of L4.end L5.end
  measures "d130" distance of L5.end L6.end
  measures "d131" distance of L5.end L8.end
  measures "d132" distance of L7.end L8.end
  measures "d133" distance of L7.end L12.end
sketch "Sketch30" plane through (0, 0, 3) normal (0, 0, 1) x (1, 0, 0)
  line L0 (213, 73) -> (209, 69)
  line L1 (213, 69) -> (209, 73)
  line L2 (213, 61) -> (209, 61)
  line L3 (209, 61) -> (209, 57)
  line L4 (209, 57) -> (213, 57)
  line L5 (213, 57) -> (213, 61)
  constraint perpendicular L0 L1
  constraint horizontal L2
  constraint vertical L3
  constraint horizontal L4
  constraint vertical L5
sketch "Sketch31" plane through (0, 0, 0) normal (0, 0, 1) x (1, 0, 0)
  line L0 (235, 85) -> (239, 85)
  line L1 (239, 85) -> (239, 73)
  line L2 (239, 73) -> (235, 73)
  line L3 (235, 73) -> (235, 85)
  dimension "d134" = 4
  dimension "d135" = 12
  constraint horizontal L0
  constraint vertical L1
  constraint horizontal L2
  constraint vertical L3
  measures "d134" distance of L0.start L0.end
  measures "d135" distance of L0.start L2.end
sketch "Sketch32" plane through (0, 0, 0) normal (1, 0, 0) x (0, 1, 0)
  circle A0 centre (-50, 25) radius 2
  circle A1 centre (-50, 25) radius 6
  line L0 (-50, 25) -> (-43, 25)
  line L1 (-43, 25) -> (-59, 25)
  dimension "d138" = 4
  dimension "d139" = 12
  constraint concentric A0 A1
  constraint coincident A0.centre A1.centre
  constraint horizontal L0
  constraint parallel L0 L1
  measures "d138" diameter of A0
  measures "d139" diameter of A1
extrude "Extrude24" add sketch "Sketch32" along normal blind 2 separate body contours A0 A1 L0 L1 picked at (-52.064, 29.1711) makes body 6
move_body "Move1" bodies 6 to x (1, 0, 0) y (0, 1, 0) z (0, 0, 1) at (0, 100, -210)
move_body "Move2" bodies 6 to x (1, 0, 0) y (0, 1, 0) z (0, 0, 1) at (214, 17, 190)
move_body "MoveFace3" bodies 6 to x (1, 0, 0) y (0, 1, 0) z (0, 0, 1) at (-4, 0, -2) on bodies 6
extrude "Extrude25" add 1 faces at (212, 64.936, 7.1711) along direction (1, 0, 0) blind 1 on bodies 6 bodies 6 2
